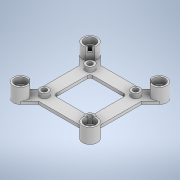
# Autodesk Inventor part: Integrated_Stepper_NEMA23_Mount
Saved by Autodesk Inventor 2021 (Build 250183000, 183)
## iProperties
Created: 2021-04-08
Part Number: Integrated_Stepper_NEMA23_Mount
Material: Generic
Document SubType Name: Modeling
Designer: Jorian Brusind
Density: 1 g/cm^3
Appearance: Default
Author: Jorian Brusind
Autodesk Inventor part; units mm, degrees
ref_plane "YZ Plane" through (0, 0, 0) normal (1, 0, 0) x (0, 1, 0)
ref_plane "XZ Plane" through (0, 0, 0) normal (0, 1, 0) x (-1, 0, 0)
ref_plane "XY Plane" through (0, 0, 0) normal (0, 0, 1) x (1, 0, 0)
sketch "Sketch1" plane through (0, 0, 0) normal (0, 1, 0) x (-1, 0, 0)
  line L0 (-21, -21) -> (21, -21)
  line L1 (21, -21) -> (21, 21)
  line L2 (21, 21) -> (-21, 21)
  line L3 (-21, 21) -> (-21, -21)
  line L4 (-21, -21) -> (21, 21) construction
  line L5 (21, -21) -> (-21, 21) construction
  circle A0 centre (15.5, 15.5) radius 1.75
  circle A1 centre (0, 0) radius 1
  circle A2 centre (-15.5, 15.5) radius 1.75
  circle A3 centre (-15.5, -15.5) radius 1.75
  circle A4 centre (15.5, -15.5) radius 1.75
  arc A5 (21.2, 15.5) -> (15.5, 21.2) centre (15.5, 15.5) ccw
  line L6 (15.5, 15.5) -> (15.5, 21.2) construction
  line L7 (15.5, 15.5) -> (21.2, 15.5) construction
  line L8 (15.5, 15.5) -> (21.2, 15.5) construction
  arc A6 (-15.5, 21.2) -> (-21.2, 15.5) centre (-15.5, 15.5) ccw
  arc A7 (-21.2, -15.5) -> (-15.5, -21.2) centre (-15.5, -15.5) ccw
  arc A8 (15.5, -21.2) -> (21.2, -15.5) centre (15.5, -15.5) ccw
  point P0 (16.9967, -21)
  point P1 (21, -16.9967)
  point P2 (21, 16.9967)
  point P3 (16.9967, 21)
  point P4 (-16.9967, 21)
  point P5 (-21, 16.9967)
  point P6 (-21, -16.9967)
  point P7 (-16.9967, -21)
  dimension "d0" = 42
  dimension "d1" = 42
  dimension "d2" = 3.5
  dimension "d3" = 5.5
  dimension "d4" = 2
  dimension "d7" = 360
  dimension "d9" = 5.7
  dimension "d10" = 90
  dimension "d11" = 90
  dimension "d14" = 360
  constraints: 18 end point, 9 centre point, 8 point on circle, 2 coincident, 2 horizontal, 2 midpoint, 2 parallel, 2 perpendicular, 1 point on line, 26 other
  measures "d0" distance of L2.end L1.end
  measures "d1" distance of L1.end L0.end
  measures "d2" diameter of A0
  measures "d3" distance from line of L1 A0.centre
  measures "d4" diameter of A1
  measures "d9" radius of A5
  measures "d10" angle of L7 L6
  measures "d11" angle of L8 L6
extrude "Extrusion1" add sketch "Sketch1" along normal blind 2 contours A7 L3 A6 L2 A5 L1 A8 L0
sketch "Sketch2" plane through (0, 2, 0) normal (0, 1, 0) x (1, 0, 0)
  line L0 (0, 0) -> (-23.5, 23.5)
  line L1 (0, 0) -> (33.234, 0) construction
  circle A0 centre (-23.5, 23.5) radius 2.25
  line L2 (-7.5, 7.5) -> (-23.5, 23.5) construction
  circle A1 centre (-15.5, 15.5) radius 1.75 projected
  line L3 (-3.9645, 11.0355) -> (-19.9645, 27.0355)
  line L4 (-27.0355, 19.9645) -> (-11.0355, 3.9645)
  arc A2 (-11.0355, 3.9645) -> (-3.9645, 11.0355) centre (-7.5, 7.5) ccw
  arc A3 (-19.9645, 27.0355) -> (-27.0355, 19.9645) centre (-23.5, 23.5) ccw
  dimension "d18" = 33.234
  dimension "d19" = 135
  dimension "d20" = 4.5
  dimension "d21" = 10
  constraints: 12 end point, 4 point on circle, 4 tangent, 3 centre point, 1 coincident, 1 equal length, 1 horizontal, 1 midpoint, 1 parallel
  measures "d18" distance of L0.start L0.end
  measures "d19" angle of L1 L0
  measures "d20" diameter of A0
  measures "d21" diameter of A3
extrude "Extrusion2" add sketch "Sketch2" against normal blind 2
pattern_circular "Circular Pattern1" count 4 over 360 about axis through (0, -10, 0) along (0, 1, 0) of "Extrusion2"
sketch "Sketch3" plane through (0, 2, 0) normal (0, 1, 0) x (1, 0, 0)
  circle A0 centre (-23.5, 23.5) radius 2.25 projected
  circle A1 centre (-23.5, 23.5) radius 3.875
  circle A2 centre (-23.5, 23.5) radius 5
  point P0 (0, 0)
  dimension "d27" = 7.75
  dimension "d28" = 10
  constraints: 2 centre point, 2 coincident
  measures "d27" diameter of A1
  measures "d28" diameter of A2
extrude "Extrusion3" add sketch "Sketch3" along normal blind 4 contours A1 | A2
sketch "Sketch4" plane through (-23.5, 6, -23.5) normal (0, 1, 0) x (1, 0, 0)
  circle A0 centre (0, 0) radius 2.25 projected
  circle A1 centre (0, 0) radius 3.875
  circle A2 centre (0, 0) radius 5
  point P0 (23.5, -23.5)
  dimension "d31" = 7.75
  dimension "d32" = 10
  constraints: 2 centre point, 2 coincident
  measures "d31" diameter of A1
  measures "d32" diameter of A2
extrude "Extrusion4" add sketch "Sketch4" along normal blind 4 contours A2
pattern_circular "Circular Pattern2" count 4 over 360 about axis through (0, 0, 0) along (0, 1, 0) of "Extrusion4", "Extrusion3"
sketch "Sketch5" plane through (0, 2, 0) normal (0, 1, 0) x (1, 0, 0)
  line L0 (22, 22) -> (-22, 22)
  line L1 (-22, 22) -> (-22, -22)
  line L2 (-22, -22) -> (22, -22)
  line L3 (22, -22) -> (22, 22)
  circle A0 centre (0, 0) radius 1 projected
  line L4 (22, 22) -> (-22, -22) construction
  line L5 (-22, 22) -> (22, -22) construction
  line L6 (-22, -22) -> (-18.4645, -18.4645)
  line L7 (-22, -22) -> (-17, -22) construction
  arc A1 (-22, -18.4645) -> (-18.4645, -22) centre (-18.4645, -18.4645) ccw
  line L8 (-18.4645, -18.4645) -> (-22, -18.4645) construction
  line L9 (-18.4645, -18.4645) -> (-18.4645, -22) construction
  arc A2 (18.4645, -22) -> (22, -18.4645) centre (18.4645, -18.4645) ccw
  arc A3 (22, 18.4645) -> (18.4645, 22) centre (18.4645, 18.4645) ccw
  arc A4 (-18.4645, 22) -> (-22, 18.4645) centre (-18.4645, 18.4645) ccw
  point P0 (22, -18.4645)
  point P1 (22, 18.4645)
  dimension "d38" = 44
  dimension "d39" = 44
  dimension "d42" = 5
  dimension "d43" = 45
  dimension "d44" = 90
  dimension "d47" = 360
  constraints: 20 end point, 8 point on circle, 4 centre point, 2 horizontal, 2 midpoint, 2 parallel, 1 coincident, 1 collinear, 1 equal length, 1 perpendicular, 1 point on line, 17 other
  measures "d38" distance of L2.end L1.end
  measures "d39" distance of L1.end L0.end
  measures "d42" distance of L1.end L6.end
  measures "d43" angle of L7 L6
  measures "d44" angle of L8 L9
extrude "Extrusion6" cut sketch "Sketch5" along normal up to surface (8 mm away) contours A3 L3 A2 L2 A1 L1 A4 L0
sketch "Sketch7" plane through (0, 2, 0) normal (0, 1, 0) x (1, 0, 0)
  line L0 (-16.9967, -21) -> (16.9967, -21) projected
  line L1 (12.5, 12.5) -> (-12.5, 12.5)
  line L2 (-12.5, 12.5) -> (-12.5, -12.5)
  line L3 (-12.5, -12.5) -> (12.5, -12.5)
  line L4 (12.5, -12.5) -> (12.5, 12.5)
  line L5 (12.5, 12.5) -> (-12.5, -12.5) construction
  line L6 (-12.5, 12.5) -> (12.5, -12.5) construction
  point P0 (0, 0)
  point P1 (-13.9289, -21)
  point P2 (13.9289, -21)
  point P3 (0, 0)
  dimension "d53" = 25
  dimension "d54" = 25
  constraints: 12 end point, 2 midpoint, 2 parallel, 1 horizontal, 1 perpendicular
  measures "d53" distance of L3.end L2.end
  measures "d54" distance of L2.end L1.end
extrude "Extrusion8" cut sketch "Sketch7" against normal through all
fillet "Fillet1" radius 2 4 edges at (-12.5, 1, -12.5) (-12.5, 1, 12.5) (12.5, 1, 12.5) (12.5, 1, -12.5)
sketch "Sketch8" plane through (0, 2, 0) normal (0, 1, 0) x (1, 0, 0)
  circle A0 centre (-15.5, 15.5) radius 1.75 projected
  circle A1 centre (-15.5, 15.5) radius 1.75
  circle A2 centre (-15.5, 15.5) radius 3
  point P0 (0, 0)
  dimension "d58" = 6
  constraints: 2 centre point, 2 coincident
  measures "d58" diameter of A2
extrude "Extrusion9" add sketch "Sketch8" along normal blind 3
pattern_circular "Circular Pattern3" count 4 over 360 about axis through (0, -10, 0) along (0, 1, 0) of "Extrusion9"
body "Solid1"
